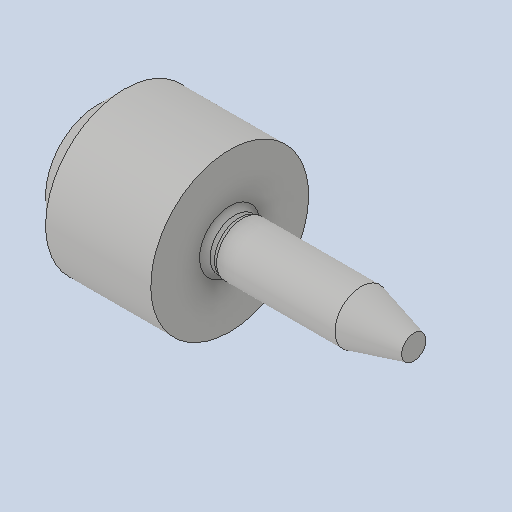
# Autodesk Inventor part: SFPSA6-P2-L5-B5
Saved by Autodesk Inventor 2024.2 (Build 282272000, 272)
## iProperties
Category: PARTsolutions
Company: MISUMI
Created: 2024-01-11
Part Number: SFPSA6-P2-L5-B5
Material: Generic
Description: FPSA, FPSPA, FPSA-R, FPSPA-R, GFPSA, GFPSPA, GFPSA-R, GFPSPA-R, BFPSA, BFPSPA, BFPSPA-R, SFPSA, SFPSPA, SFPSA-R, SFPSPA-R, HFPSA, HFPSPA, HFPSA-R, HFPSPA-R, CFPSA, CFPSPA, CFPSA-R, CFPSPA-R, LFPSA, LFPSPA, LFPSA-R, LFPSPA-R-Locating Pins - Small Head, Tapered - Press Fit - P, L, B Configurable - Round Type
Vendor: MISUMI
Document SubType Name: Modeling
Designer: psAdmin
Manufacturer: MISUMI
Mass: 0.152133 g
Surface Area: 1.76671 cm^2
Volume: 0.152133 cm^3
Density: 1 g/cm^3
Appearance: PSOLRGB-175-175-175
Catalog Web Link: https://jp.misumi-ec.com/vona2/detail/110300559670/?ProductCode=SFPSA6-P2-L5-B5
PSOL_IDENT_0: {$CADENAS_DATA/23d-libs/misumi/metric/14_locating_pins/fpsa.prj},447 {VTYP=3D},{NB=SFPSA6-P2.00-L5-B
PSOL_IDENT_1: 5.0},{LINA=SFPSA6-P2.00-L5-B5.0},{NN=FPSA, FPSPA, FPSA-R, FPSPA-R, GFPSA, GFPSPA, GFPSA-R, GFPSPA-R,
PSOL_IDENT_2: BFPSA, BFPSPA, BFPSPA-R, SFPSA, SFPSPA, SFPSA-R, SFPSPA-R, HFPSA, HFPSPA, HFPSA-R, HFPSPA-R, CFPSA,
PSOL_IDENT_3: CFPSPA, CFPSA-R, CFPSPA-R, LFPSA, LFPSPA, LFPSA-R, LFPSPA-R},{DATE=29.05.2023 02:21:04},{GEOMDATE=3
PSOL_IDENT_4: 0.06.2020 05:26:20},{VERSION=},{LINEID=340},{WBVAR=MAT,ST,HARD,DTOL,TSS,P,L,BS,ALT1,TC,ALT2},{WBNUME
PSOL_IDENT_5: RIC=P,L,BS,TC}  {NB=SFPSA6-P2.00-L5-B5.0},{LINA=SFPSA6-P2.00-L5-B5.0},{KT=DUMMY},{PN=SFPSA6-P2.00-L5
PSOL_IDENT_6: -B5.0},{TYPE=SFPS},{MAT=SUS304},{MATALG= 'SKS3' , 'SKS3 Equivalent' , 'SUS304' , 'SUS304' , 'SUS440C'
PSOL_IDENT_7: , 'SUS440C Equivalent' , 'SUS316' , '316 Stainless Steel' },{ST=-},{STALG= '-' , '-' , 'HCP' , 'Har
PSOL_IDENT_8: d Chrome Plating' },{HARD=-},{HARDALG= '-' , '-' },{DTOL=A},{DTOLALG= 'A' , 'SA(m6)' , 'PA' , 'SPA(p
PSOL_IDENT_9: 6)' },{TSS=},{TSSALG= '' , '-' },{D=6},{P=2.00},{PALG= [ 2 : 6 / 0.01 ] },{PMIN=2},{PMAX=6},{L=5},{L
PSOL_IDENT_10: ALG= [ 5 : 17 / 1 ] },{LMIN=5},{LMAX=17},{BS=5.0},{B=5.0},{BALG= [ 2 : 15 / 0.1 ] },{BMIN=2},{BMAX=1
PSOL_IDENT_11: 5},{C=1.0},{MM=2.0},{LL=1},{R1=0.0},{R2=0},{ALPHA1=60},{ALT1=},{ALT1ALG= '' , 'Not applicable' },{TC=
PSOL_IDENT_12: 0},{TCALG=0},{TCMINT=3},{TCMAXT=9},{TCMAXF1=5},{TCMAXF2=1},{TCMAXF=1},{TCMAX=1},{ALT2=},{ALT2ALG= ''
PSOL_IDENT_13: , 'w/o RC (Spherical Tip)' , '-RC' , 'with RC (Spherical Tip)' },{RC=0.5},{ALT1PN=},{ALT2PN=},{PPN=
PSOL_IDENT_14: 2.00},{BPN=5.0},{PAA=0.5},{PDD=1.90},{SALG=1}
NB: SFPSA6-P2.00-L5-B5.0
NN: FPSA, FPSPA, FPSA-R, FPSPA-R, GFPSA, GFPSPA, GFPSA-R, GFPSPA-R, BFPSA, BFPSPA, BFPSPA-R, SFPSA, SFPSPA, SFPSA-R, SFPSPA-R, HFPSA, HFPSPA, HFPSA-R, HFPSPA-R, CFPSA, CFPSPA, CFPSA-R, CFPSPA-R, LFPSA, LFPSPA, LFPSA-R, LFPSPA-R
NT: Locating Pins - Small Head, Tapered - Press Fit - P, L, B Configurable - Round Type
NBSYN: $PN.
LINA: SFPSA6-P2.00-L5-B5.0
CATALOG: Misumi
PN: SFPSA6-P2.00-L5-B5.0
MAT: SUS304
ST: -
HARD: -
DTOL: SA(m6)
TSS: -
D: 6
P: 2
L: 5
BS: 5
C: 1
MM: 2
LL: 1
ALT1: Not applicable
TC: 0
ALT2: w/o RC (Spherical Tip)
SUPPLIER: MISUMI
ARTICLENO: SFPSA6-P2.00-L5-B5.0
BOMINFO: SFPSA6-P2.00-L5-B5.0
CREATOR: CADENAS GmbH
Title: SFPSA6-P2.00-L5-B5.0
Author: Cadenas PARTsolutions
Comments: Locating Pins - Small Head, Tapered - Press Fit - P, L, B Configurable - Round Type
Autodesk Inventor part; units mm, degrees
ref_plane "YZ Plane" through (0, 0, 0) normal (1, 0, 0) x (0, 1, 0)
ref_plane "XZ Plane" through (0, 0, 0) normal (0, 1, 0) x (-1, 0, 0)
ref_plane "XY Plane" through (0, 0, 0) normal (0, 0, 1) x (1, 0, 0)
sketch "Sketch_1" plane through (0, 0, 0) normal (0, 0, 1) x (1, 0, 0)
  line L0 (0, 0) -> (-5, 0)
  line L1 (-5, 0) -> (-5, 2)
  line L2 (-5, 2) -> (-4, 3)
  line L3 (-4, 3) -> (0.5, 3)
  line L4 (0.5, 3) -> (0.5, 0)
  line L5 (0.5, 0) -> (-5, 0)
  constraints: 12 end point
revolve "Revolution1" add sketch "Sketch_1" angle 360 about axis through (0, 0, 0) along (1, 0, 0)
sketch "Sketch_2" plane through (0, 0, 0) normal (0, 0, 1) x (1, 0, 0)
  line L0 (7, 0) -> (0, 0)
  line L1 (0, 0) -> (0, 1)
  line L2 (0, 1) -> (5, 1)
  line L3 (5, 1) -> (7, 0.4641)
  line L4 (7, 0.4641) -> (7, 0)
  line L5 (7, 0) -> (0, 0)
  constraints: 12 end point
revolve "Revolution2" add sketch "Sketch_2" angle 360 about axis through (7, 0, 0) along (1, 0, 0)
sketch "Sketch_13" plane through (0, 0, 0) normal (0, 0, 1) x (1, 0, 0)
  line L0 (50, 0) -> (-50, 0)
  line L1 (0, 6) -> (0, 1.15)
  arc A0 (0, 1.15) -> (0.2, 0.95) centre (0.2, 1.15) ccw
  line L2 (0.2, 0.95) -> (0.3677, 0.95)
  arc A1 (0.3677, 0.95) -> (0.5, 1) centre (0.3677, 1.15) ccw
  line L3 (0.5, 1) -> (0.5, 6)
  line L4 (0.5, 6) -> (0, 6)
  constraints: 10 end point, 4 point on circle, 2 centre point
revolve "Revolution3" cut sketch "Sketch_13" angle 360 about axis through (50, 0, 0) along (1, 0, 0)
body "Solid1"
